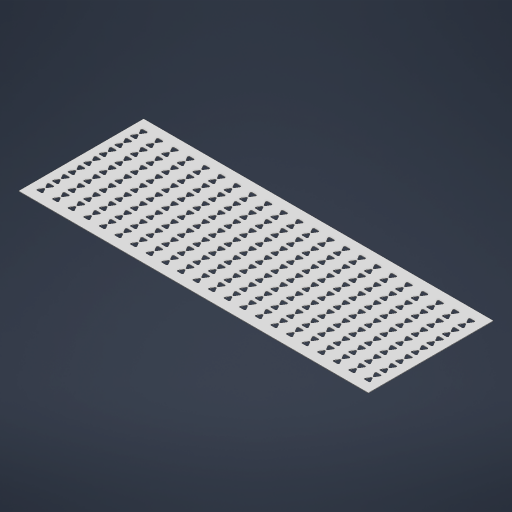
# Autodesk Inventor part: BellyPan
Saved by Autodesk Inventor 2023 (Build 270158000, 158)
## iProperties
Created: 2022-04-16
Part Number: BellyPan
Material: Generic
Document SubType Name: Modeling
Designer: timmy
Density: 1 g/cm^3
Appearance: Default
Author: timmy
Autodesk Inventor part; units mm, degrees
(part 1 of 4)
ref_plane "YZ Plane" through (0, 0, 0) normal (1, 0, 0) x (0, 1, 0)
ref_plane "XZ Plane" through (0, 0, 0) normal (0, 1, 0) x (-1, 0, 0)
ref_plane "XY Plane" through (0, 0, 0) normal (0, 0, 1) x (1, 0, 0)
sketch "Sketch1" plane through (0, 0, 0) normal (0, 1, 0) x (-1, 0, 0)
  line L0 (0, 0) -> (1219.2, 0)
  line L1 (1219.2, 0) -> (1219.2, -436.0164)
  line L2 (1219.2, -436.0164) -> (0, -436.0164)
  line L3 (0, -436.0164) -> (0, 0)
  dimension "d0" = 1219.2
  dimension "d1" = 436.0164
  constraints: 8 end point, 2 parallel, 1 horizontal, 1 perpendicular
  measures "d0" distance of L1.end L2.end
  measures "d1" distance of L0.end L1.end
extrude "Extrusion1" add sketch "Sketch1" along normal blind 1.5875
sketch "Sketch2" plane through (0, 1.5875, 0) normal (0, 1, 0) x (1, 0, 0)
  line L0 (0, 436.0164) -> (-1219.2, 436.0164) projected
  line L1 (-1219.2, 436.0164) -> (-1219.2, 0) projected
  line L2 (-1219.2, 0) -> (0, 0) projected
  line L3 (0, 0) -> (0, 436.0164) projected
  line L4 (-1193.8, 410.6164) -> (-1193.8, 25.4)
  line L5 (-25.4, 410.6164) -> (-1193.8, 410.6164)
  line L6 (-1188.4934, 33.8582) -> (-1174.092, 33.8582)
  line L7 (-1171.3423, 38.6207) -> (-1178.5431, 51.0927)
  line L8 (-1184.0423, 51.0927) -> (-1191.2431, 38.6207)
  arc A0 (-1191.2431, 38.6207) -> (-1188.4934, 33.8582) centre (-1188.4934, 37.0332) ccw
  arc A1 (-1174.092, 33.8582) -> (-1171.3423, 38.6207) centre (-1174.092, 37.0332) ccw
  arc A2 (-1178.5431, 51.0927) -> (-1184.0423, 51.0927) centre (-1181.2927, 49.5052) ccw
  line L9 (-1188.3007, 76.2) -> (-1173.8993, 76.2)
  line L10 (-1171.1496, 71.4375) -> (-1178.3504, 58.9655)
  line L11 (-1183.8496, 58.9655) -> (-1191.0504, 71.4375)
  arc A3 (-1188.3007, 76.2) -> (-1191.0504, 71.4375) centre (-1188.3007, 73.025) ccw
  arc A4 (-1171.1496, 71.4375) -> (-1173.8993, 76.2) centre (-1173.8993, 73.025) ccw
  arc A5 (-1183.8496, 58.9655) -> (-1178.3504, 58.9655) centre (-1181.1, 60.553) ccw
  line L12 (-1183.8496, 113.3215) -> (-1191.0504, 125.7935)
  arc A6 (-1171.1496, 125.7935) -> (-1173.8993, 130.556) centre (-1173.8993, 127.381) ccw
  arc A7 (-1188.3007, 130.556) -> (-1191.0504, 125.7935) centre (-1188.3007, 127.381) ccw
  arc A8 (-1183.8496, 113.3215) -> (-1178.3504, 113.3215) centre (-1181.1, 114.909) ccw
  line L13 (-1171.1496, 125.7935) -> (-1178.3504, 113.3215)
  line L14 (-1188.3007, 130.556) -> (-1173.8993, 130.556)
  arc A9 (-1178.5431, 105.4487) -> (-1184.0423, 105.4487) centre (-1181.2927, 103.8612) ccw
  line L15 (-1171.3423, 92.9767) -> (-1178.5431, 105.4487)
  line L16 (-1184.0423, 105.4487) -> (-1191.2431, 92.9767)
  arc A10 (-1191.2431, 92.9767) -> (-1188.4934, 88.2142) centre (-1188.4934, 91.3892) ccw
  line L17 (-1188.4934, 88.2142) -> (-1174.092, 88.2142)
  arc A11 (-1174.092, 88.2142) -> (-1171.3423, 92.9767) centre (-1174.092, 91.3892) ccw
  line L18 (-1183.8496, 167.6775) -> (-1191.0504, 180.1495)
  arc A12 (-1171.1496, 180.1495) -> (-1173.8993, 184.912) centre (-1173.8993, 181.737) ccw
  arc A13 (-1188.3007, 184.912) -> (-1191.0504, 180.1495) centre (-1188.3007, 181.737) ccw
  arc A14 (-1183.8496, 167.6775) -> (-1178.3504, 167.6775) centre (-1181.1, 169.265) ccw
  line L19 (-1171.1496, 180.1495) -> (-1178.3504, 167.6775)
  line L20 (-1188.3007, 184.912) -> (-1173.8993, 184.912)
  arc A15 (-1178.5431, 159.8047) -> (-1184.0423, 159.8047) centre (-1181.2927, 158.2172) ccw
  line L21 (-1171.3423, 147.3327) -> (-1178.5431, 159.8047)
  line L22 (-1184.0423, 159.8047) -> (-1191.2431, 147.3327)
  arc A16 (-1191.2431, 147.3327) -> (-1188.4934, 142.5702) centre (-1188.4934, 145.7452) ccw
  line L23 (-1188.4934, 142.5702) -> (-1174.092, 142.5702)
  arc A17 (-1174.092, 142.5702) -> (-1171.3423, 147.3327) centre (-1174.092, 145.7452) ccw
  line L24 (-1183.8496, 222.0335) -> (-1191.0504, 234.5055)
  arc A18 (-1171.1496, 234.5055) -> (-1173.8993, 239.268) centre (-1173.8993, 236.093) ccw
  arc A19 (-1188.3007, 239.268) -> (-1191.0504, 234.5055) centre (-1188.3007, 236.093) ccw
  arc A20 (-1183.8496, 222.0335) -> (-1178.3504, 222.0335) centre (-1181.1, 223.621) ccw
  line L25 (-1171.1496, 234.5055) -> (-1178.3504, 222.0335)
  line L26 (-1188.3007, 239.268) -> (-1173.8993, 239.268)
  arc A21 (-1178.5431, 214.1607) -> (-1184.0423, 214.1607) centre (-1181.2927, 212.5732) ccw
  line L27 (-1171.3423, 201.6887) -> (-1178.5431, 214.1607)
  line L28 (-1184.0423, 214.1607) -> (-1191.2431, 201.6887)
  arc A22 (-1191.2431, 201.6887) -> (-1188.4934, 196.9262) centre (-1188.4934, 200.1012) ccw
  line L29 (-1188.4934, 196.9262) -> (-1174.092, 196.9262)
  arc A23 (-1174.092, 196.9262) -> (-1171.3423, 201.6887) centre (-1174.092, 200.1012) ccw
  line L30 (-1183.8496, 276.3895) -> (-1191.0504, 288.8615)
  arc A24 (-1171.1496, 288.8615) -> (-1173.8993, 293.624) centre (-1173.8993, 290.449) ccw
  arc A25 (-1188.3007, 293.624) -> (-1191.0504, 288.8615) centre (-1188.3007, 290.449) ccw
  arc A26 (-1183.8496, 276.3895) -> (-1178.3504, 276.3895) centre (-1181.1, 277.977) ccw
  line L31 (-1171.1496, 288.8615) -> (-1178.3504, 276.3895)
  line L32 (-1188.3007, 293.624) -> (-1173.8993, 293.624)
  arc A27 (-1178.5431, 268.5167) -> (-1184.0423, 268.5167) centre (-1181.2927, 266.9292) ccw
  line L33 (-1171.3423, 256.0447) -> (-1178.5431, 268.5167)
  line L34 (-1184.0423, 268.5167) -> (-1191.2431, 256.0447)
  arc A28 (-1191.2431, 256.0447) -> (-1188.4934, 251.2822) centre (-1188.4934, 254.4572) ccw
  line L35 (-1188.4934, 251.2822) -> (-1174.092, 251.2822)
  arc A29 (-1174.092, 251.2822) -> (-1171.3423, 256.0447) centre (-1174.092, 254.4572) ccw
  line L36 (-1183.8496, 330.7455) -> (-1191.0504, 343.2175)
  arc A30 (-1171.1496, 343.2175) -> (-1173.8993, 347.98) centre (-1173.8993, 344.805) ccw
  arc A31 (-1188.3007, 347.98) -> (-1191.0504, 343.2175) centre (-1188.3007, 344.805) ccw
  arc A32 (-1183.8496, 330.7455) -> (-1178.3504, 330.7455) centre (-1181.1, 332.333) ccw
  line L37 (-1171.1496, 343.2175) -> (-1178.3504, 330.7455)
  line L38 (-1188.3007, 347.98) -> (-1173.8993, 347.98)
  arc A33 (-1178.5431, 322.8727) -> (-1184.0423, 322.8727) centre (-1181.2927, 321.2852) ccw
  line L39 (-1171.3423, 310.4007) -> (-1178.5431, 322.8727)
  line L40 (-1184.0423, 322.8727) -> (-1191.2431, 310.4007)
  arc A34 (-1191.2431, 310.4007) -> (-1188.4934, 305.6382) centre (-1188.4934, 308.8132) ccw
  line L41 (-1188.4934, 305.6382) -> (-1174.092, 305.6382)
  arc A35 (-1174.092, 305.6382) -> (-1171.3423, 310.4007) centre (-1174.092, 308.8132) ccw
  line L42 (-1183.8496, 385.1015) -> (-1191.0504, 397.5735)
  arc A36 (-1171.1496, 397.5735) -> (-1173.8993, 402.336) centre (-1173.8993, 399.161) ccw
  arc A37 (-1188.3007, 402.336) -> (-1191.0504, 397.5735) centre (-1188.3007, 399.161) ccw
  arc A38 (-1183.8496, 385.1015) -> (-1178.3504, 385.1015) centre (-1181.1, 386.689) ccw
  line L43 (-1171.1496, 397.5735) -> (-1178.3504, 385.1015)
  line L44 (-1188.3007, 402.336) -> (-1173.8993, 402.336)
  arc A39 (-1178.5431, 377.2287) -> (-1184.0423, 377.2287) centre (-1181.2927, 375.6412) ccw
  line L45 (-1171.3423, 364.7567) -> (-1178.5431, 377.2287)
  line L46 (-1184.0423, 377.2287) -> (-1191.2431, 364.7567)
  arc A40 (-1191.2431, 364.7567) -> (-1188.4934, 359.9942) centre (-1188.4934, 363.1692) ccw
  line L47 (-1188.4934, 359.9942) -> (-1174.092, 359.9942)
  arc A41 (-1174.092, 359.9942) -> (-1171.3423, 364.7567) centre (-1174.092, 363.1692) ccw
  line L48 (-1129.4936, 58.9655) -> (-1136.6944, 71.4375)
  arc A42 (-1116.7936, 71.4375) -> (-1119.5433, 76.2) centre (-1119.5433, 73.025) ccw
  arc A43 (-1133.9447, 76.2) -> (-1136.6944, 71.4375) centre (-1133.9447, 73.025) ccw
  arc A44 (-1129.4936, 58.9655) -> (-1123.9944, 58.9655) centre (-1126.744, 60.553) ccw
  line L49 (-1116.7936, 71.4375) -> (-1123.9944, 58.9655)
  line L50 (-1133.9447, 76.2) -> (-1119.5433, 76.2)
  arc A45 (-1124.1871, 51.0927) -> (-1129.6863, 51.0927) centre (-1126.9367, 49.5052) ccw
  line L51 (-1116.9863, 38.6207) -> (-1124.1871, 51.0927)
  line L52 (-1129.6863, 51.0927) -> (-1136.8871, 38.6207)
  arc A46 (-1136.8871, 38.6207) -> (-1134.1374, 33.8582) centre (-1134.1374, 37.0332) ccw
  line L53 (-1134.1374, 33.8582) -> (-1119.736, 33.8582)
  arc A47 (-1119.736, 33.8582) -> (-1116.9863, 38.6207) centre (-1119.736, 37.0332) ccw
  line L54 (-1129.4936, 113.3215) -> (-1136.6944, 125.7935)
  arc A48 (-1116.7936, 125.7935) -> (-1119.5433, 130.556) centre (-1119.5433, 127.381) ccw
  arc A49 (-1133.9447, 130.556) -> (-1136.6944, 125.7935) centre (-1133.9447, 127.381) ccw
  arc A50 (-1129.4936, 113.3215) -> (-1123.9944, 113.3215) centre (-1126.744, 114.909) ccw
  line L55 (-1116.7936, 125.7935) -> (-1123.9944, 113.3215)
  line L56 (-1133.9447, 130.556) -> (-1119.5433, 130.556)
  arc A51 (-1124.1871, 105.4487) -> (-1129.6863, 105.4487) centre (-1126.9367, 103.8612) ccw
  line L57 (-1116.9863, 92.9767) -> (-1124.1871, 105.4487)
  line L58 (-1129.6863, 105.4487) -> (-1136.8871, 92.9767)
  arc A52 (-1136.8871, 92.9767) -> (-1134.1374, 88.2142) centre (-1134.1374, 91.3892) ccw
  line L59 (-1134.1374, 88.2142) -> (-1119.736, 88.2142)
  arc A53 (-1119.736, 88.2142) -> (-1116.9863, 92.9767) centre (-1119.736, 91.3892) ccw
  line L60 (-1129.4936, 167.6775) -> (-1136.6944, 180.1495)
  arc A54 (-1116.7936, 180.1495) -> (-1119.5433, 184.912) centre (-1119.5433, 181.737) ccw
  arc A55 (-1133.9447, 184.912) -> (-1136.6944, 180.1495) centre (-1133.9447, 181.737) ccw
  arc A56 (-1129.4936, 167.6775) -> (-1123.9944, 167.6775) centre (-1126.744, 169.265) ccw
  line L61 (-1116.7936, 180.1495) -> (-1123.9944, 167.6775)
  line L62 (-1133.9447, 184.912) -> (-1119.5433, 184.912)
  arc A57 (-1124.1871, 159.8047) -> (-1129.6863, 159.8047) centre (-1126.9367, 158.2172) ccw
  line L63 (-1116.9863, 147.3327) -> (-1124.1871, 159.8047)
  line L64 (-1129.6863, 159.8047) -> (-1136.8871, 147.3327)
  arc A58 (-1136.8871, 147.3327) -> (-1134.1374, 142.5702) centre (-1134.1374, 145.7452) ccw
  line L65 (-1134.1374, 142.5702) -> (-1119.736, 142.5702)
  arc A59 (-1119.736, 142.5702) -> (-1116.9863, 147.3327) centre (-1119.736, 145.7452) ccw
  line L66 (-1129.4936, 222.0335) -> (-1136.6944, 234.5055)
  arc A60 (-1116.7936, 234.5055) -> (-1119.5433, 239.268) centre (-1119.5433, 236.093) ccw
  arc A61 (-1133.9447, 239.268) -> (-1136.6944, 234.5055) centre (-1133.9447, 236.093) ccw
  arc A62 (-1129.4936, 222.0335) -> (-1123.9944, 222.0335) centre (-1126.744, 223.621) ccw
  line L67 (-1116.7936, 234.5055) -> (-1123.9944, 222.0335)
  line L68 (-1133.9447, 239.268) -> (-1119.5433, 239.268)
  arc A63 (-1124.1871, 214.1607) -> (-1129.6863, 214.1607) centre (-1126.9367, 212.5732) ccw
  line L69 (-1116.9863, 201.6887) -> (-1124.1871, 214.1607)
  line L70 (-1129.6863, 214.1607) -> (-1136.8871, 201.6887)
  arc A64 (-1136.8871, 201.6887) -> (-1134.1374, 196.9262) centre (-1134.1374, 200.1012) ccw
  line L71 (-1134.1374, 196.9262) -> (-1119.736, 196.9262)
  arc A65 (-1119.736, 196.9262) -> (-1116.9863, 201.6887) centre (-1119.736, 200.1012) ccw
  line L72 (-1129.4936, 276.3895) -> (-1136.6944, 288.8615)
  arc A66 (-1116.7936, 288.8615) -> (-1119.5433, 293.624) centre (-1119.5433, 290.449) ccw
  arc A67 (-1133.9447, 293.624) -> (-1136.6944, 288.8615) centre (-1133.9447, 290.449) ccw
  arc A68 (-1129.4936, 276.3895) -> (-1123.9944, 276.3895) centre (-1126.744, 277.977) ccw
  line L73 (-1116.7936, 288.8615) -> (-1123.9944, 276.3895)
  line L74 (-1133.9447, 293.624) -> (-1119.5433, 293.624)
  arc A69 (-1124.1871, 268.5167) -> (-1129.6863, 268.5167) centre (-1126.9367, 266.9292) ccw
  line L75 (-1116.9863, 256.0447) -> (-1124.1871, 268.5167)
  line L76 (-1129.6863, 268.5167) -> (-1136.8871, 256.0447)
  arc A70 (-1136.8871, 256.0447) -> (-1134.1374, 251.2822) centre (-1134.1374, 254.4572) ccw
  line L77 (-1134.1374, 251.2822) -> (-1119.736, 251.2822)
  arc A71 (-1119.736, 251.2822) -> (-1116.9863, 256.0447) centre (-1119.736, 254.4572) ccw
  line L78 (-1129.4936, 330.7455) -> (-1136.6944, 343.2175)
  arc A72 (-1116.7936, 343.2175) -> (-1119.5433, 347.98) centre (-1119.5433, 344.805) ccw
  arc A73 (-1133.9447, 347.98) -> (-1136.6944, 343.2175) centre (-1133.9447, 344.805) ccw
  arc A74 (-1129.4936, 330.7455) -> (-1123.9944, 330.7455) centre (-1126.744, 332.333) ccw
  line L79 (-1116.7936, 343.2175) -> (-1123.9944, 330.7455)
  line L80 (-1133.9447, 347.98) -> (-1119.5433, 347.98)
  arc A75 (-1124.1871, 322.8727) -> (-1129.6863, 322.8727) centre (-1126.9367, 321.2852) ccw
  line L81 (-1116.9863, 310.4007) -> (-1124.1871, 322.8727)
  line L82 (-1129.6863, 322.8727) -> (-1136.8871, 310.4007)
  arc A76 (-1136.8871, 310.4007) -> (-1134.1374, 305.6382) centre (-1134.1374, 308.8132) ccw
  line L83 (-1134.1374, 305.6382) -> (-1119.736, 305.6382)
  arc A77 (-1119.736, 305.6382) -> (-1116.9863, 310.4007) centre (-1119.736, 308.8132) ccw
  line L84 (-1129.4936, 385.1015) -> (-1136.6944, 397.5735)
  arc A78 (-1116.7936, 397.5735) -> (-1119.5433, 402.336) centre (-1119.5433, 399.161) ccw
  arc A79 (-1133.9447, 402.336) -> (-1136.6944, 397.5735) centre (-1133.9447, 399.161) ccw
  arc A80 (-1129.4936, 385.1015) -> (-1123.9944, 385.1015) centre (-1126.744, 386.689) ccw
  line L85 (-1116.7936, 397.5735) -> (-1123.9944, 385.1015)
  line L86 (-1133.9447, 402.336) -> (-1119.5433, 402.336)
  arc A81 (-1124.1871, 377.2287) -> (-1129.6863, 377.2287) centre (-1126.9367, 375.6412) ccw
  line L87 (-1116.9863, 364.7567) -> (-1124.1871, 377.2287)
  line L88 (-1129.6863, 377.2287) -> (-1136.8871, 364.7567)
  arc A82 (-1136.8871, 364.7567) -> (-1134.1374, 359.9942) centre (-1134.1374, 363.1692) ccw
  line L89 (-1134.1374, 359.9942) -> (-1119.736, 359.9942)
  arc A83 (-1119.736, 359.9942) -> (-1116.9863, 364.7567) centre (-1119.736, 363.1692) ccw
  line L90 (-1075.1376, 58.9655) -> (-1082.3384, 71.4375)
  arc A84 (-1062.4376, 71.4375) -> (-1065.1873, 76.2) centre (-1065.1873, 73.025) ccw
  arc A85 (-1079.5887, 76.2) -> (-1082.3384, 71.4375) centre (-1079.5887, 73.025) ccw
  arc A86 (-1075.1376, 58.9655) -> (-1069.6384, 58.9655) centre (-1072.388, 60.553) ccw
  line L91 (-1062.4376, 71.4375) -> (-1069.6384, 58.9655)
  line L92 (-1079.5887, 76.2) -> (-1065.1873, 76.2)
  arc A87 (-1069.8311, 51.0927) -> (-1075.3303, 51.0927) centre (-1072.5807, 49.5052) ccw
  line L93 (-1062.6303, 38.6207) -> (-1069.8311, 51.0927)
  line L94 (-1075.3303, 51.0927) -> (-1082.5311, 38.6207)
  arc A88 (-1082.5311, 38.6207) -> (-1079.7814, 33.8582) centre (-1079.7814, 37.0332) ccw
  line L95 (-1079.7814, 33.8582) -> (-1065.38, 33.8582)
  arc A89 (-1065.38, 33.8582) -> (-1062.6303, 38.6207) centre (-1065.38, 37.0332) ccw
  line L96 (-1075.1376, 113.3215) -> (-1082.3384, 125.7935)
  arc A90 (-1062.4376, 125.7935) -> (-1065.1873, 130.556) centre (-1065.1873, 127.381) ccw
  arc A91 (-1079.5887, 130.556) -> (-1082.3384, 125.7935) centre (-1079.5887, 127.381) ccw
  arc A92 (-1075.1376, 113.3215) -> (-1069.6384, 113.3215) centre (-1072.388, 114.909) ccw
  line L97 (-1062.4376, 125.7935) -> (-1069.6384, 113.3215)
  line L98 (-1079.5887, 130.556) -> (-1065.1873, 130.556)
  arc A93 (-1069.8311, 105.4487) -> (-1075.3303, 105.4487) centre (-1072.5807, 103.8612) ccw
  line L99 (-1062.6303, 92.9767) -> (-1069.8311, 105.4487)
  line L100 (-1075.3303, 105.4487) -> (-1082.5311, 92.9767)
  arc A94 (-1082.5311, 92.9767) -> (-1079.7814, 88.2142) centre (-1079.7814, 91.3892) ccw
  line L101 (-1079.7814, 88.2142) -> (-1065.38, 88.2142)
  arc A95 (-1065.38, 88.2142) -> (-1062.6303, 92.9767) centre (-1065.38, 91.3892) ccw
  line L102 (-1075.1376, 167.6775) -> (-1082.3384, 180.1495)
  arc A96 (-1062.4376, 180.1495) -> (-1065.1873, 184.912) centre (-1065.1873, 181.737) ccw
  arc A97 (-1079.5887, 184.912) -> (-1082.3384, 180.1495) centre (-1079.5887, 181.737) ccw
  arc A98 (-1075.1376, 167.6775) -> (-1069.6384, 167.6775) centre (-1072.388, 169.265) ccw
  line L103 (-1062.4376, 180.1495) -> (-1069.6384, 167.6775)
  line L104 (-1079.5887, 184.912) -> (-1065.1873, 184.912)
  arc A99 (-1069.8311, 159.8047) -> (-1075.3303, 159.8047) centre (-1072.5807, 158.2172) ccw
  line L105 (-1062.6303, 147.3327) -> (-1069.8311, 159.8047)
  line L106 (-1075.3303, 159.8047) -> (-1082.5311, 147.3327)
  arc A100 (-1082.5311, 147.3327) -> (-1079.7814, 142.5702) centre (-1079.7814, 145.7452) ccw
  line L107 (-1079.7814, 142.5702) -> (-1065.38, 142.5702)
  arc A101 (-1065.38, 142.5702) -> (-1062.6303, 147.3327) centre (-1065.38, 145.7452) ccw
  line L108 (-1075.1376, 222.0335) -> (-1082.3384, 234.5055)
  arc A102 (-1062.4376, 234.5055) -> (-1065.1873, 239.268) centre (-1065.1873, 236.093) ccw
  arc A103 (-1079.5887, 239.268) -> (-1082.3384, 234.5055) centre (-1079.5887, 236.093) ccw
  arc A104 (-1075.1376, 222.0335) -> (-1069.6384, 222.0335) centre (-1072.388, 223.621) ccw
  line L109 (-1062.4376, 234.5055) -> (-1069.6384, 222.0335)
  line L110 (-1079.5887, 239.268) -> (-1065.1873, 239.268)
  arc A105 (-1069.8311, 214.1607) -> (-1075.3303, 214.1607) centre (-1072.5807, 212.5732) ccw
  line L111 (-1062.6303, 201.6887) -> (-1069.8311, 214.1607)
  line L112 (-1075.3303, 214.1607) -> (-1082.5311, 201.6887)
  arc A106 (-1082.5311, 201.6887) -> (-1079.7814, 196.9262) centre (-1079.7814, 200.1012) ccw
  line L113 (-1079.7814, 196.9262) -> (-1065.38, 196.9262)
  arc A107 (-1065.38, 196.9262) -> (-1062.6303, 201.6887) centre (-1065.38, 200.1012) ccw
  line L114 (-1075.1376, 276.3895) -> (-1082.3384, 288.8615)
  arc A108 (-1062.4376, 288.8615) -> (-1065.1873, 293.624) centre (-1065.1873, 290.449) ccw
  arc A109 (-1079.5887, 293.624) -> (-1082.3384, 288.8615) centre (-1079.5887, 290.449) ccw
  arc A110 (-1075.1376, 276.3895) -> (-1069.6384, 276.3895) centre (-1072.388, 277.977) ccw
  line L115 (-1062.4376, 288.8615) -> (-1069.6384, 276.3895)
  line L116 (-1079.5887, 293.624) -> (-1065.1873, 293.624)
  arc A111 (-1069.8311, 268.5167) -> (-1075.3303, 268.5167) centre (-1072.5807, 266.9292) ccw
  line L117 (-1062.6303, 256.0447) -> (-1069.8311, 268.5167)
  line L118 (-1075.3303, 268.5167) -> (-1082.5311, 256.0447)
  arc A112 (-1082.5311, 256.0447) -> (-1079.7814, 251.2822) centre (-1079.7814, 254.4572) ccw
  line L119 (-1079.7814, 251.2822) -> (-1065.38, 251.2822)
  arc A113 (-1065.38, 251.2822) -> (-1062.6303, 256.0447) centre (-1065.38, 254.4572) ccw
  line L120 (-1075.1376, 330.7455) -> (-1082.3384, 343.2175)
  arc A114 (-1062.4376, 343.2175) -> (-1065.1873, 347.98) centre (-1065.1873, 344.805) ccw
  arc A115 (-1079.5887, 347.98) -> (-1082.3384, 343.2175) centre (-1079.5887, 344.805) ccw
  arc A116 (-1075.1376, 330.7455) -> (-1069.6384, 330.7455) centre (-1072.388, 332.333) ccw
  line L121 (-1062.4376, 343.2175) -> (-1069.6384, 330.7455)
  line L122 (-1079.5887, 347.98) -> (-1065.1873, 347.98)
  arc A117 (-1069.8311, 322.8727) -> (-1075.3303, 322.8727) centre (-1072.5807, 321.2852) ccw
  line L123 (-1062.6303, 310.4007) -> (-1069.8311, 322.8727)
  line L124 (-1075.3303, 322.8727) -> (-1082.5311, 310.4007)
  arc A118 (-1082.5311, 310.4007) -> (-1079.7814, 305.6382) centre (-1079.7814, 308.8132) ccw
  line L125 (-1079.7814, 305.6382) -> (-1065.38, 305.6382)
  arc A119 (-1065.38, 305.6382) -> (-1062.6303, 310.4007) centre (-1065.38, 308.8132) ccw
  line L126 (-1075.1376, 385.1015) -> (-1082.3384, 397.5735)
  arc A120 (-1062.4376, 397.5735) -> (-1065.1873, 402.336) centre (-1065.1873, 399.161) ccw
  arc A121 (-1079.5887, 402.336) -> (-1082.3384, 397.5735) centre (-1079.5887, 399.161) ccw
  arc A122 (-1075.1376, 385.1015) -> (-1069.6384, 385.1015) centre (-1072.388, 386.689) ccw
  line L127 (-1062.4376, 397.5735) -> (-1069.6384, 385.1015)
  line L128 (-1079.5887, 402.336) -> (-1065.1873, 402.336)
  arc A123 (-1069.8311, 377.2287) -> (-1075.3303, 377.2287) centre (-1072.5807, 375.6412) ccw
  line L129 (-1062.6303, 364.7567) -> (-1069.8311, 377.2287)
  line L130 (-1075.3303, 377.2287) -> (-1082.5311, 364.7567)
  arc A124 (-1082.5311, 364.7567) -> (-1079.7814, 359.9942) centre (-1079.7814, 363.1692) ccw
  line L131 (-1079.7814, 359.9942) -> (-1065.38, 359.9942)
  arc A125 (-1065.38, 359.9942) -> (-1062.6303, 364.7567) centre (-1065.38, 363.1692) ccw
  line L132 (-1020.7816, 58.9655) -> (-1027.9824, 71.4375)
  arc A126 (-1008.0816, 71.4375) -> (-1010.8313, 76.2) centre (-1010.8313, 73.025) ccw
  arc A127 (-1025.2327, 76.2) -> (-1027.9824, 71.4375) centre (-1025.2327, 73.025) ccw
  arc A128 (-1020.7816, 58.9655) -> (-1015.2824, 58.9655) centre (-1018.032, 60.553) ccw
  line L133 (-1008.0816, 71.4375) -> (-1015.2824, 58.9655)
  line L134 (-1025.2327, 76.2) -> (-1010.8313, 76.2)
  arc A129 (-1015.4751, 51.0927) -> (-1020.9743, 51.0927) centre (-1018.2247, 49.5052) ccw
  line L135 (-1008.2743, 38.6207) -> (-1015.4751, 51.0927)
  line L136 (-1020.9743, 51.0927) -> (-1028.1751, 38.6207)
  arc A130 (-1028.1751, 38.6207) -> (-1025.4254, 33.8582) centre (-1025.4254, 37.0332) ccw
  line L137 (-1025.4254, 33.8582) -> (-1011.024, 33.8582)
  arc A131 (-1011.024, 33.8582) -> (-1008.2743, 38.6207) centre (-1011.024, 37.0332) ccw
  line L138 (-1020.7816, 113.3215) -> (-1027.9824, 125.7935)
  arc A132 (-1008.0816, 125.7935) -> (-1010.8313, 130.556) centre (-1010.8313, 127.381) ccw
  arc A133 (-1025.2327, 130.556) -> (-1027.9824, 125.7935) centre (-1025.2327, 127.381) ccw
  arc A134 (-1020.7816, 113.3215) -> (-1015.2824, 113.3215) centre (-1018.032, 114.909) ccw
  line L139 (-1008.0816, 125.7935) -> (-1015.2824, 113.3215)
  line L140 (-1025.2327, 130.556) -> (-1010.8313, 130.556)
  arc A135 (-1015.4751, 105.4487) -> (-1020.9743, 105.4487) centre (-1018.2247, 103.8612) ccw
  line L141 (-1008.2743, 92.9767) -> (-1015.4751, 105.4487)
  line L142 (-1020.9743, 105.4487) -> (-1028.1751, 92.9767)
  arc A136 (-1028.1751, 92.9767) -> (-1025.4254, 88.2142) centre (-1025.4254, 91.3892) ccw
  line L143 (-1025.4254, 88.2142) -> (-1011.024, 88.2142)
  arc A137 (-1011.024, 88.2142) -> (-1008.2743, 92.9767) centre (-1011.024, 91.3892) ccw
  line L144 (-1020.7816, 167.6775) -> (-1027.9824, 180.1495)
  arc A138 (-1008.0816, 180.1495) -> (-1010.8313, 184.912) centre (-1010.8313, 181.737) ccw
  arc A139 (-1025.2327, 184.912) -> (-1027.9824, 180.1495) centre (-1025.2327, 181.737) ccw
  arc A140 (-1020.7816, 167.6775) -> (-1015.2824, 167.6775) centre (-1018.032, 169.265) ccw
  line L145 (-1008.0816, 180.1495) -> (-1015.2824, 167.6775)
  line L146 (-1025.2327, 184.912) -> (-1010.8313, 184.912)
  arc A141 (-1015.4751, 159.8047) -> (-1020.9743, 159.8047) centre (-1018.2247, 158.2172) ccw
  line L147 (-1008.2743, 147.3327) -> (-1015.4751, 159.8047)
  line L148 (-1020.9743, 159.8047) -> (-1028.1751, 147.3327)
  arc A142 (-1028.1751, 147.3327) -> (-1025.4254, 142.5702) centre (-1025.4254, 145.7452) ccw
  line L149 (-1025.4254, 142.5702) -> (-1011.024, 142.5702)
  arc A143 (-1011.024, 142.5702) -> (-1008.2743, 147.3327) centre (-1011.024, 145.7452) ccw
  line L150 (-1020.7816, 222.0335) -> (-1027.9824, 234.5055)
  arc A144 (-1008.0816, 234.5055) -> (-1010.8313, 239.268) centre (-1010.8313, 236.093) ccw
  arc A145 (-1025.2327, 239.268) -> (-1027.9824, 234.5055) centre (-1025.2327, 236.093) ccw
  arc A146 (-1020.7816, 222.0335) -> (-1015.2824, 222.0335) centre (-1018.032, 223.621) ccw
  line L151 (-1008.0816, 234.5055) -> (-1015.2824, 222.0335)
  line L152 (-1025.2327, 239.268) -> (-1010.8313, 239.268)
  arc A147 (-1015.4751, 214.1607) -> (-1020.9743, 214.1607) centre (-1018.2247, 212.5732) ccw
  line L153 (-1008.2743, 201.6887) -> (-1015.4751, 214.1607)
  line L154 (-1020.9743, 214.1607) -> (-1028.1751, 201.6887)
  arc A148 (-1028.1751, 201.6887) -> (-1025.4254, 196.9262) centre (-1025.4254, 200.1012) ccw
  line L155 (-1025.4254, 196.9262) -> (-1011.024, 196.9262)
  arc A149 (-1011.024, 196.9262) -> (-1008.2743, 201.6887) centre (-1011.024, 200.1012) ccw
  line L156 (-1020.7816, 276.3895) -> (-1027.9824, 288.8615)
  arc A150 (-1008.0816, 288.8615) -> (-1010.8313, 293.624) centre (-1010.8313, 290.449) ccw
  arc A151 (-1025.2327, 293.624) -> (-1027.9824, 288.8615) centre (-1025.2327, 290.449) ccw
  arc A152 (-1020.7816, 276.3895) -> (-1015.2824, 276.3895) centre (-1018.032, 277.977) ccw
  line L157 (-1008.0816, 288.8615) -> (-1015.2824, 276.3895)
  line L158 (-1025.2327, 293.624) -> (-1010.8313, 293.624)
  arc A153 (-1015.4751, 268.5167) -> (-1020.9743, 268.5167) centre (-1018.2247, 266.9292) ccw
  line L159 (-1008.2743, 256.0447) -> (-1015.4751, 268.5167)
  line L160 (-1020.9743, 268.5167) -> (-1028.1751, 256.0447)
  arc A154 (-1028.1751, 256.0447) -> (-1025.4254, 251.2822) centre (-1025.4254, 254.4572) ccw
  line L161 (-1025.4254, 251.2822) -> (-1011.024, 251.2822)
  arc A155 (-1011.024, 251.2822) -> (-1008.2743, 256.0447) centre (-1011.024, 254.4572) ccw
  line L162 (-1020.7816, 330.7455) -> (-1027.9824, 343.2175)
  arc A156 (-1008.0816, 343.2175) -> (-1010.8313, 347.98) centre (-1010.8313, 344.805) ccw
  arc A157 (-1025.2327, 347.98) -> (-1027.9824, 343.2175) centre (-1025.2327, 344.805) ccw
  arc A158 (-1020.7816, 330.7455) -> (-1015.2824, 330.7455) centre (-1018.032, 332.333) ccw
  line L163 (-1008.0816, 343.2175) -> (-1015.2824, 330.7455)
  line L164 (-1025.2327, 347.98) -> (-1010.8313, 347.98)
  arc A159 (-1015.4751, 322.8727) -> (-1020.9743, 322.8727) centre (-1018.2247, 321.2852) ccw
  line L165 (-1008.2743, 310.4007) -> (-1015.4751, 322.8727)
  line L166 (-1020.9743, 322.8727) -> (-1028.1751, 310.4007)
  arc A160 (-1028.1751, 310.4007) -> (-1025.4254, 305.6382) centre (-1025.4254, 308.8132) ccw
  line L167 (-1025.4254, 305.6382) -> (-1011.024, 305.6382)
  arc A161 (-1011.024, 305.6382) -> (-1008.2743, 310.4007) centre (-1011.024, 308.8132) ccw
  line L168 (-1020.7816, 385.1015) -> (-1027.9824, 397.5735)
  arc A162 (-1008.0816, 397.5735) -> (-1010.8313, 402.336) centre (-1010.8313, 399.161) ccw
  arc A163 (-1025.2327, 402.336) -> (-1027.9824, 397.5735) centre (-1025.2327, 399.161) ccw
  arc A164 (-1020.7816, 385.1015) -> (-1015.2824, 385.1015) centre (-1018.032, 386.689) ccw
  line L169 (-1008.0816, 397.5735) -> (-1015.2824, 385.1015)
  line L170 (-1025.2327, 402.336) -> (-1010.8313, 402.336)
  arc A165 (-1015.4751, 377.2287) -> (-1020.9743, 377.2287) centre (-1018.2247, 375.6412) ccw
  line L171 (-1008.2743, 364.7567) -> (-1015.4751, 377.2287)
  line L172 (-1020.9743, 377.2287) -> (-1028.1751, 364.7567)
  arc A166 (-1028.1751, 364.7567) -> (-1025.4254, 359.9942) centre (-1025.4254, 363.1692) ccw
  line L173 (-1025.4254, 359.9942) -> (-1011.024, 359.9942)
  arc A167 (-1011.024, 359.9942) -> (-1008.2743, 364.7567) centre (-1011.024, 363.1692) ccw
  line L174 (-966.4256, 58.9655) -> (-973.6264, 71.4375)
  arc A168 (-953.7256, 71.4375) -> (-956.4753, 76.2) centre (-956.4753, 73.025) ccw
  arc A169 (-970.8767, 76.2) -> (-973.6264, 71.4375) centre (-970.8767, 73.025) ccw
  arc A170 (-966.4256, 58.9655) -> (-960.9264, 58.9655) centre (-963.676, 60.553) ccw
  line L175 (-953.7256, 71.4375) -> (-960.9264, 58.9655)
  line L176 (-970.8767, 76.2) -> (-956.4753, 76.2)
  arc A171 (-961.1191, 51.0927) -> (-966.6183, 51.0927) centre (-963.8687, 49.5052) ccw
  line L177 (-953.9183, 38.6207) -> (-961.1191, 51.0927)
  line L178 (-966.6183, 51.0927) -> (-973.8191, 38.6207)
  arc A172 (-973.8191, 38.6207) -> (-971.0694, 33.8582) centre (-971.0694, 37.0332) ccw
  line L179 (-971.0694, 33.8582) -> (-956.668, 33.8582)
  arc A173 (-956.668, 33.8582) -> (-953.9183, 38.6207) centre (-956.668, 37.0332) ccw
  line L180 (-966.4256, 113.3215) -> (-973.6264, 125.7935)
  arc A174 (-953.7256, 125.7935) -> (-956.4753, 130.556) centre (-956.4753, 127.381) ccw
  arc A175 (-970.8767, 130.556) -> (-973.6264, 125.7935) centre (-970.8767, 127.381) ccw
  arc A176 (-966.4256, 113.3215) -> (-960.9264, 113.3215) centre (-963.676, 114.909) ccw
  line L181 (-953.7256, 125.7935) -> (-960.9264, 113.3215)
  line L182 (-970.8767, 130.556) -> (-956.4753, 130.556)
  arc A177 (-961.1191, 105.4487) -> (-966.6183, 105.4487) centre (-963.8687, 103.8612) ccw
  line L183 (-953.9183, 92.9767) -> (-961.1191, 105.4487)
  line L184 (-966.6183, 105.4487) -> (-973.8191, 92.9767)
  arc A178 (-973.8191, 92.9767) -> (-971.0694, 88.2142) centre (-971.0694, 91.3892) ccw
  line L185 (-971.0694, 88.2142) -> (-956.668, 88.2142)
  arc A179 (-956.668, 88.2142) -> (-953.9183, 92.9767) centre (-956.668, 91.3892) ccw
  line L186 (-966.4256, 167.6775) -> (-973.6264, 180.1495)
  arc A180 (-953.7256, 180.1495) -> (-956.4753, 184.912) centre (-956.4753, 181.737) ccw
  arc A181 (-970.8767, 184.912) -> (-973.6264, 180.1495) centre (-970.8767, 181.737) ccw
  arc A182 (-966.4256, 167.6775) -> (-960.9264, 167.6775) centre (-963.676, 169.265) ccw
  line L187 (-953.7256, 180.1495) -> (-960.9264, 167.6775)
  line L188 (-970.8767, 184.912) -> (-956.4753, 184.912)
  arc A183 (-961.1191, 159.8047) -> (-966.6183, 159.8047) centre (-963.8687, 158.2172) ccw
  line L189 (-953.9183, 147.3327) -> (-961.1191, 159.8047)
  line L190 (-966.6183, 159.8047) -> (-973.8191, 147.3327)
  arc A184 (-973.8191, 147.3327) -> (-971.0694, 142.5702) centre (-971.0694, 145.7452) ccw
  line L191 (-971.0694, 142.5702) -> (-956.668, 142.5702)
  arc A185 (-956.668, 142.5702) -> (-953.9183, 147.3327) centre (-956.668, 145.7452) ccw
  line L192 (-966.4256, 222.0335) -> (-973.6264, 234.5055)
  arc A186 (-953.7256, 234.5055) -> (-956.4753, 239.268) centre (-956.4753, 236.093) ccw
  arc A187 (-970.8767, 239.268) -> (-973.6264, 234.5055) centre (-970.8767, 236.093) ccw
  arc A188 (-966.4256, 222.0335) -> (-960.9264, 222.0335) centre (-963.676, 223.621) ccw
  line L193 (-953.7256, 234.5055) -> (-960.9264, 222.0335)
  line L194 (-970.8767, 239.268) -> (-956.4753, 239.268)
  arc A189 (-961.1191, 214.1607) -> (-966.6183, 214.1607) centre (-963.8687, 212.5732) ccw
  line L195 (-953.9183, 201.6887) -> (-961.1191, 214.1607)
  line L196 (-966.6183, 214.1607) -> (-973.8191, 201.6887)
  arc A190 (-973.8191, 201.6887) -> (-971.0694, 196.9262) centre (-971.0694, 200.1012) ccw
  line L197 (-971.0694, 196.9262) -> (-956.668, 196.9262)
  arc A191 (-956.668, 196.9262) -> (-953.9183, 201.6887) centre (-956.668, 200.1012) ccw
  line L198 (-966.4256, 276.3895) -> (-973.6264, 288.8615)
  arc A192 (-953.7256, 288.8615) -> (-956.4753, 293.624) centre (-956.4753, 290.449) ccw
  arc A193 (-970.8767, 293.624) -> (-973.6264, 288.8615) centre (-970.8767, 290.449) ccw
  arc A194 (-966.4256, 276.3895) -> (-960.9264, 276.3895) centre (-963.676, 277.977) ccw
  line L199 (-953.7256, 288.8615) -> (-960.9264, 276.3895)
  line L200 (-970.8767, 293.624) -> (-956.4753, 293.624)
  arc A195 (-961.1191, 268.5167) -> (-966.6183, 268.5167) centre (-963.8687, 266.9292) ccw
  line L201 (-953.9183, 256.0447) -> (-961.1191, 268.5167)
  line L202 (-966.6183, 268.5167) -> (-973.8191, 256.0447)
  arc A196 (-973.8191, 256.0447) -> (-971.0694, 251.2822) centre (-971.0694, 254.4572) ccw
  line L203 (-971.0694, 251.2822) -> (-956.668, 251.2822)
  arc A197 (-956.668, 251.2822) -> (-953.9183, 256.0447) centre (-956.668, 254.4572) ccw
  line L204 (-966.4256, 330.7455) -> (-973.6264, 343.2175)
  arc A198 (-953.7256, 343.2175) -> (-956.4753, 347.98) centre (-956.4753, 344.805) ccw
  arc A199 (-970.8767, 347.98) -> (-973.6264, 343.2175) centre (-970.8767, 344.805) ccw
  arc A200 (-966.4256, 330.7455) -> (-960.9264, 330.7455) centre (-963.676, 332.333) ccw
  line L205 (-953.7256, 343.2175) -> (-960.9264, 330.7455)
  line L206 (-970.8767, 347.98) -> (-956.4753, 347.98)
  arc A201 (-961.1191, 322.8727) -> (-966.6183, 322.8727) centre (-963.8687, 321.2852) ccw
  line L207 (-953.9183, 310.4007) -> (-961.1191, 322.8727)
  line L208 (-966.6183, 322.8727) -> (-973.8191, 310.4007)
  arc A202 (-973.8191, 310.4007) -> (-971.0694, 305.6382) centre (-971.0694, 308.8132) ccw
  line L209 (-971.0694, 305.6382) -> (-956.668, 305.6382)
  arc A203 (-956.668, 305.6382) -> (-953.9183, 310.4007) centre (-956.668, 308.8132) ccw
  line L210 (-966.4256, 385.1015) -> (-973.6264, 397.5735)
  arc A204 (-953.7256, 397.5735) -> (-956.4753, 402.336) centre (-956.4753, 399.161) ccw
  arc A205 (-970.8767, 402.336) -> (-973.6264, 397.5735) centre (-970.8767, 399.161) ccw
  arc A206 (-966.4256, 385.1015) -> (-960.9264, 385.1015) centre (-963.676, 386.689) ccw
  line L211 (-953.7256, 397.5735) -> (-960.9264, 385.1015)
  line L212 (-970.8767, 402.336) -> (-956.4753, 402.336)
  arc A207 (-961.1191, 377.2287) -> (-966.6183, 377.2287) centre (-963.8687, 375.6412) ccw
  line L213 (-953.9183, 364.7567) -> (-961.1191, 377.2287)
  line L214 (-966.6183, 377.2287) -> (-973.8191, 364.7567)
  arc A208 (-973.8191, 364.7567) -> (-971.0694, 359.9942) centre (-971.0694, 363.1692) ccw
  line L215 (-971.0694, 359.9942) -> (-956.668, 359.9942)
  arc A209 (-956.668, 359.9942) -> (-953.9183, 364.7567) centre (-956.668, 363.1692) ccw
  line L216 (-912.0696, 58.9655) -> (-919.2704, 71.4375)
  arc A210 (-899.3696, 71.4375) -> (-902.1193, 76.2) centre (-902.1193, 73.025) ccw
  arc A211 (-916.5207, 76.2) -> (-919.2704, 71.4375) centre (-916.5207, 73.025) ccw
  arc A212 (-912.0696, 58.9655) -> (-906.5704, 58.9655) centre (-909.32, 60.553) ccw
  line L217 (-899.3696, 71.4375) -> (-906.5704, 58.9655)
  line L218 (-916.5207, 76.2) -> (-902.1193, 76.2)
  arc A213 (-906.7631, 51.0927) -> (-912.2623, 51.0927) centre (-909.5127, 49.5052) ccw
  line L219 (-899.5623, 38.6207) -> (-906.7631, 51.0927)
  line L220 (-912.2623, 51.0927) -> (-919.4631, 38.6207)
  arc A214 (-919.4631, 38.6207) -> (-916.7134, 33.8582) centre (-916.7134, 37.0332) ccw
  line L221 (-916.7134, 33.8582) -> (-902.312, 33.8582)
  arc A215 (-902.312, 33.8582) -> (-899.5623, 38.6207) centre (-902.312, 37.0332) ccw
  line L222 (-912.0696, 113.3215) -> (-919.2704, 125.7935)
  arc A216 (-899.3696, 125.7935) -> (-902.1193, 130.556) centre (-902.1193, 127.381) ccw
  arc A217 (-916.5207, 130.556) -> (-919.2704, 125.7935) centre (-916.5207, 127.381) ccw
  arc A218 (-912.0696, 113.3215) -> (-906.5704, 113.3215) centre (-909.32, 114.909) ccw
  line L223 (-899.3696, 125.7935) -> (-906.5704, 113.3215)
  line L224 (-916.5207, 130.556) -> (-902.1193, 130.556)
  arc A219 (-906.7631, 105.4487) -> (-912.2623, 105.4487) centre (-909.5127, 103.8612) ccw
  line L225 (-899.5623, 92.9767) -> (-906.7631, 105.4487)
  line L226 (-912.2623, 105.4487) -> (-919.4631, 92.9767)
  arc A220 (-919.4631, 92.9767) -> (-916.7134, 88.2142) centre (-916.7134, 91.3892) ccw
  line L227 (-916.7134, 88.2142) -> (-902.312, 88.2142)
  arc A221 (-902.312, 88.2142) -> (-899.5623, 92.9767) centre (-902.312, 91.3892) ccw
  line L228 (-912.0696, 167.6775) -> (-919.2704, 180.1495)
  arc A222 (-899.3696, 180.1495) -> (-902.1193, 184.912) centre (-902.1193, 181.737) ccw
  arc A223 (-916.5207, 184.912) -> (-919.2704, 180.1495) centre (-916.5207, 181.737) ccw
  arc A224 (-912.0696, 167.6775) -> (-906.5704, 167.6775) centre (-909.32, 169.265) ccw
  line L229 (-899.3696, 180.1495) -> (-906.5704, 167.6775)
  line L230 (-916.5207, 184.912) -> (-902.1193, 184.912)
  arc A225 (-906.7631, 159.8047) -> (-912.2623, 159.8047) centre (-909.5127, 158.2172) ccw
  line L231 (-899.5623, 147.3327) -> (-906.7631, 159.8047)
  line L232 (-912.2623, 159.8047) -> (-919.4631, 147.3327)
  arc A226 (-919.4631, 147.3327) -> (-916.7134, 142.5702) centre (-916.7134, 145.7452) ccw
  line L233 (-916.7134, 142.5702) -> (-902.312, 142.5702)
  arc A227 (-902.312, 142.5702) -> (-899.5623, 147.3327) centre (-902.312, 145.7452) ccw
  line L234 (-912.0696, 222.0335) -> (-919.2704, 234.5055)
  arc A228 (-899.3696, 234.5055) -> (-902.1193, 239.268) centre (-902.1193, 236.093) ccw
  arc A229 (-916.5207, 239.268) -> (-919.2704, 234.5055) centre (-916.5207, 236.093) ccw
  arc A230 (-912.0696, 222.0335) -> (-906.5704, 222.0335) centre (-909.32, 223.621) ccw
  line L235 (-899.3696, 234.5055) -> (-906.5704, 222.0335)
  line L236 (-916.5207, 239.268) -> (-902.1193, 239.268)
  arc A231 (-906.7631, 214.1607) -> (-912.2623, 214.1607) centre (-909.5127, 212.5732) ccw
  line L237 (-899.5623, 201.6887) -> (-906.7631, 214.1607)
  line L238 (-912.2623, 214.1607) -> (-919.4631, 201.6887)
  arc A232 (-919.4631, 201.6887) -> (-916.7134, 196.9262) centre (-916.7134, 200.1012) ccw
  line L239 (-916.7134, 196.9262) -> (-902.312, 196.9262)
  arc A233 (-902.312, 196.9262) -> (-899.5623, 201.6887) centre (-902.312, 200.1012) ccw
  line L240 (-912.0696, 276.3895) -> (-919.2704, 288.8615)
  arc A234 (-899.3696, 288.8615) -> (-902.1193, 293.624) centre (-902.1193, 290.449) ccw
  arc A235 (-916.5207, 293.624) -> (-919.2704, 288.8615) centre (-916.5207, 290.449) ccw
  arc A236 (-912.0696, 276.3895) -> (-906.5704, 276.3895) centre (-909.32, 277.977) ccw
  line L241 (-899.3696, 288.8615) -> (-906.5704, 276.3895)
  line L242 (-916.5207, 293.624) -> (-902.1193, 293.624)
  arc A237 (-906.7631, 268.5167) -> (-912.2623, 268.5167) centre (-909.5127, 266.9292) ccw
  line L243 (-899.5623, 256.0447) -> (-906.7631, 268.5167)
  line L244 (-912.2623, 268.5167) -> (-919.4631, 256.0447)
  arc A238 (-919.4631, 256.0447) -> (-916.7134, 251.2822) centre (-916.7134, 254.4572) ccw
  line L245 (-916.7134, 251.2822) -> (-902.312, 251.2822)
  arc A239 (-902.312, 251.2822) -> (-899.5623, 256.0447) centre (-902.312, 254.4572) ccw
  line L246 (-912.0696, 330.7455) -> (-919.2704, 343.2175)
  arc A240 (-899.3696, 343.2175) -> (-902.1193, 347.98) centre (-902.1193, 344.805) ccw
  arc A241 (-916.5207, 347.98) -> (-919.2704, 343.2175) centre (-916.5207, 344.805) ccw
  arc A242 (-912.0696, 330.7455) -> (-906.5704, 330.7455) centre (-909.32, 332.333) ccw
  line L247 (-899.3696, 343.2175) -> (-906.5704, 330.7455)
  line L248 (-916.5207, 347.98) -> (-902.1193, 347.98)
  arc A243 (-906.7631, 322.8727) -> (-912.2623, 322.8727) centre (-909.5127, 321.2852) ccw
  line L249 (-899.5623, 310.4007) -> (-906.7631, 322.8727)
  line L250 (-912.2623, 322.8727) -> (-919.4631, 310.4007)
  arc A244 (-919.4631, 310.4007) -> (-916.7134, 305.6382) centre (-916.7134, 308.8132) ccw
  line L251 (-916.7134, 305.6382) -> (-902.312, 305.6382)
  arc A245 (-902.312, 305.6382) -> (-899.5623, 310.4007) centre (-902.312, 308.8132) ccw
  line L252 (-912.0696, 385.1015) -> (-919.2704, 397.5735)
  arc A246 (-899.3696, 397.5735) -> (-902.1193, 402.336) centre (-902.1193, 399.161) ccw
  arc A247 (-916.5207, 402.336) -> (-919.2704, 397.5735) centre (-916.5207, 399.161) ccw
  arc A248 (-912.0696, 385.1015) -> (-906.5704, 385.1015) centre (-909.32, 386.689) ccw
  line L253 (-899.3696, 397.5735) -> (-906.5704, 385.1015)
  line L254 (-916.5207, 402.336) -> (-902.1193, 402.336)
  arc A249 (-906.7631, 377.2287) -> (-912.2623, 377.2287) centre (-909.5127, 375.6412) ccw
  line L255 (-899.5623, 364.7567) -> (-906.7631, 377.2287)
  line L256 (-912.2623, 377.2287) -> (-919.4631, 364.7567)
  arc A250 (-919.4631, 364.7567) -> (-916.7134, 359.9942) centre (-916.7134, 363.1692) ccw
  line L257 (-916.7134, 359.9942) -> (-902.312, 359.9942)
  arc A251 (-902.312, 359.9942) -> (-899.5623, 364.7567) centre (-902.312, 363.1692) ccw
  line L258 (-857.7136, 58.9655) -> (-864.9144, 71.4375)
  arc A252 (-845.0136, 71.4375) -> (-847.7633, 76.2) centre (-847.7633, 73.025) ccw
  arc A253 (-862.1647, 76.2) -> (-864.9144, 71.4375) centre (-862.1647, 73.025) ccw
  arc A254 (-857.7136, 58.9655) -> (-852.2144, 58.9655) centre (-854.964, 60.553) ccw
  line L259 (-845.0136, 71.4375) -> (-852.2144, 58.9655)
  line L260 (-862.1647, 76.2) -> (-847.7633, 76.2)
  arc A255 (-852.4071, 51.0927) -> (-857.9063, 51.0927) centre (-855.1567, 49.5052) ccw
  line L261 (-845.2063, 38.6207) -> (-852.4071, 51.0927)
  line L262 (-857.9063, 51.0927) -> (-865.1071, 38.6207)
  arc A256 (-865.1071, 38.6207) -> (-862.3574, 33.8582) centre (-862.3574, 37.0332) ccw
  line L263 (-862.3574, 33.8582) -> (-847.956, 33.8582)
  arc A257 (-847.956, 33.8582) -> (-845.2063, 38.6207) centre (-847.956, 37.0332) ccw
  line L264 (-857.7136, 113.3215) -> (-864.9144, 125.7935)
  arc A258 (-845.0136, 125.7935) -> (-847.7633, 130.556) centre (-847.7633, 127.381) ccw
  arc A259 (-862.1647, 130.556) -> (-864.9144, 125.7935) centre (-862.1647, 127.381) ccw
  arc A260 (-857.7136, 113.3215) -> (-852.2144, 113.3215) centre (-854.964, 114.909) ccw
  line L265 (-845.0136, 125.7935) -> (-852.2144, 113.3215)
  line L266 (-862.1647, 130.556) -> (-847.7633, 130.556)
  arc A261 (-852.4071, 105.4487) -> (-857.9063, 105.4487) centre (-855.1567, 103.8612) ccw
  line L267 (-845.2063, 92.9767) -> (-852.4071, 105.4487)
  line L268 (-857.9063, 105.4487) -> (-865.1071, 92.9767)
  arc A262 (-865.1071, 92.9767) -> (-862.3574, 88.2142) centre (-862.3574, 91.3892) ccw
  line L269 (-862.3574, 88.2142) -> (-847.956, 88.2142)
  arc A263 (-847.956, 88.2142) -> (-845.2063, 92.9767) centre (-847.956, 91.3892) ccw
  line L270 (-857.7136, 167.6775) -> (-864.9144, 180.1495)
  arc A264 (-845.0136, 180.1495) -> (-847.7633, 184.912) centre (-847.7633, 181.737) ccw
  arc A265 (-862.1647, 184.912) -> (-864.9144, 180.1495) centre (-862.1647, 181.737) ccw
  arc A266 (-857.7136, 167.6775) -> (-852.2144, 167.6775) centre (-854.964, 169.265) ccw
  line L271 (-845.0136, 180.1495) -> (-852.2144, 167.6775)
  line L272 (-862.1647, 184.912) -> (-847.7633, 184.912)
  arc A267 (-852.4071, 159.8047) -> (-857.9063, 159.8047) centre (-855.1567, 158.2172) ccw
  line L273 (-845.2063, 147.3327) -> (-852.4071, 159.8047)
  line L274 (-857.9063, 159.8047) -> (-865.1071, 147.3327)
  arc A268 (-865.1071, 147.3327) -> (-862.3574, 142.5702) centre (-862.3574, 145.7452) ccw
  line L275 (-862.3574, 142.5702) -> (-847.956, 142.5702)
  arc A269 (-847.956, 142.5702) -> (-845.2063, 147.3327) centre (-847.956, 145.7452) ccw
  line L276 (-857.7136, 222.0335) -> (-864.9144, 234.5055)
  arc A270 (-845.0136, 234.5055) -> (-847.7633, 239.268) centre (-847.7633, 236.093) ccw
  arc A271 (-862.1647, 239.268) -> (-864.9144, 234.5055) centre (-862.1647, 236.093) ccw
  arc A272 (-857.7136, 222.0335) -> (-852.2144, 222.0335) centre (-854.964, 223.621) ccw
  line L277 (-845.0136, 234.5055) -> (-852.2144, 222.0335)
  line L278 (-862.1647, 239.268) -> (-847.7633, 239.268)
  arc A273 (-852.4071, 214.1607) -> (-857.9063, 214.1607) centre (-855.1567, 212.5732) ccw
  line L279 (-845.2063, 201.6887) -> (-852.4071, 214.1607)
  line L280 (-857.9063, 214.1607) -> (-865.1071, 201.6887)
  arc A274 (-865.1071, 201.6887) -> (-862.3574, 196.9262) centre (-862.3574, 200.1012) ccw
  line L281 (-862.3574, 196.9262) -> (-847.956, 196.9262)
  arc A275 (-847.956, 196.9262) -> (-845.2063, 201.6887) centre (-847.956, 200.1012) ccw
  line L282 (-857.7136, 276.3895) -> (-864.9144, 288.8615)
  arc A276 (-845.0136, 288.8615) -> (-847.7633, 293.624) centre (-847.7633, 290.449) ccw
  arc A277 (-862.1647, 293.624) -> (-864.9144, 288.8615) centre (-862.1647, 290.449) ccw
  arc A278 (-857.7136, 276.3895) -> (-852.2144, 276.3895) centre (-854.964, 277.977) ccw
  line L283 (-845.0136, 288.8615) -> (-852.2144, 276.3895)
  line L284 (-862.1647, 293.624) -> (-847.7633, 293.624)
  arc A279 (-852.4071, 268.5167) -> (-857.9063, 268.5167) centre (-855.1567, 266.9292) ccw
  line L285 (-845.2063, 256.0447) -> (-852.4071, 268.5167)
  line L286 (-857.9063, 268.5167) -> (-865.1071, 256.0447)
  arc A280 (-865.1071, 256.0447) -> (-862.3574, 251.2822) centre (-862.3574, 254.4572) ccw
  line L287 (-862.3574, 251.2822) -> (-847.956, 251.2822)
  arc A281 (-847.956, 251.2822) -> (-845.2063, 256.0447) centre (-847.956, 254.4572) ccw
  line L288 (-857.7136, 330.7455) -> (-864.9144, 343.2175)
  arc A282 (-845.0136, 343.2175) -> (-847.7633, 347.98) centre (-847.7633, 344.805) ccw
  arc A283 (-862.1647, 347.98) -> (-864.9144, 343.2175) centre (-862.1647, 344.805) ccw
  arc A284 (-857.7136, 330.7455) -> (-852.2144, 330.7455) centre (-854.964, 332.333) ccw
  line L289 (-845.0136, 343.2175) -> (-852.2144, 330.7455)
  line L290 (-862.1647, 347.98) -> (-847.7633, 347.98)
  arc A285 (-852.4071, 322.8727) -> (-857.9063, 322.8727) centre (-855.1567, 321.2852) ccw
  line L291 (-845.2063, 310.4007) -> (-852.4071, 322.8727)
  line L292 (-857.9063, 322.8727) -> (-865.1071, 310.4007)
  arc A286 (-865.1071, 310.4007) -> (-862.3574, 305.6382) centre (-862.3574, 308.8132) ccw
  line L293 (-862.3574, 305.6382) -> (-847.956, 305.6382)
  arc A287 (-847.956, 305.6382) -> (-845.2063, 310.4007) centre (-847.956, 308.8132) ccw
  line L294 (-857.7136, 385.1015) -> (-864.9144, 397.5735)
  arc A288 (-845.0136, 397.5735) -> (-847.7633, 402.336) centre (-847.7633, 399.161) ccw
  arc A289 (-862.1647, 402.336) -> (-864.9144, 397.5735) centre (-862.1647, 399.161) ccw
  arc A290 (-857.7136, 385.1015) -> (-852.2144, 385.1015) centre (-854.964, 386.689) ccw
  line L295 (-845.0136, 397.5735) -> (-852.2144, 385.1015)
  line L296 (-862.1647, 402.336) -> (-847.7633, 402.336)
  arc A291 (-852.4071, 377.2287) -> (-857.9063, 377.2287) centre (-855.1567, 375.6412) ccw
  line L297 (-845.2063, 364.7567) -> (-852.4071, 377.2287)
  line L298 (-857.9063, 377.2287) -> (-865.1071, 364.7567)
  arc A292 (-865.1071, 364.7567) -> (-862.3574, 359.9942) centre (-862.3574, 363.1692) ccw
  line L299 (-862.3574, 359.9942) -> (-847.956, 359.9942)
  arc A293 (-847.956, 359.9942) -> (-845.2063, 364.7567) centre (-847.956, 363.1692) ccw
  line L300 (-803.3576, 58.9655) -> (-810.5584, 71.4375)
  arc A294 (-790.6576, 71.4375) -> (-793.4073, 76.2) centre (-793.4073, 73.025) ccw
  arc A295 (-807.8087, 76.2) -> (-810.5584, 71.4375) centre (-807.8087, 73.025) ccw
  arc A296 (-803.3576, 58.9655) -> (-797.8584, 58.9655) centre (-800.608, 60.553) ccw
  line L301 (-790.6576, 71.4375) -> (-797.8584, 58.9655)
  line L302 (-807.8087, 76.2) -> (-793.4073, 76.2)
  arc A297 (-798.0511, 51.0927) -> (-803.5503, 51.0927) centre (-800.8007, 49.5052) ccw
  line L303 (-790.8503, 38.6207) -> (-798.0511, 51.0927)
  line L304 (-803.5503, 51.0927) -> (-810.7511, 38.6207)
  arc A298 (-810.7511, 38.6207) -> (-808.0014, 33.8582) centre (-808.0014, 37.0332) ccw
  line L305 (-808.0014, 33.8582) -> (-793.6, 33.8582)
  arc A299 (-793.6, 33.8582) -> (-790.8503, 38.6207) centre (-793.6, 37.0332) ccw
  line L306 (-803.3576, 113.3215) -> (-810.5584, 125.7935)
  arc A300 (-790.6576, 125.7935) -> (-793.4073, 130.556) centre (-793.4073, 127.381) ccw
  arc A301 (-807.8087, 130.556) -> (-810.5584, 125.7935) centre (-807.8087, 127.381) ccw
  arc A302 (-803.3576, 113.3215) -> (-797.8584, 113.3215) centre (-800.608, 114.909) ccw
  line L307 (-790.6576, 125.7935) -> (-797.8584, 113.3215)
  line L308 (-807.8087, 130.556) -> (-793.4073, 130.556)
  arc A303 (-798.0511, 105.4487) -> (-803.5503, 105.4487) centre (-800.8007, 103.8612) ccw
  line L309 (-790.8503, 92.9767) -> (-798.0511, 105.4487)
  line L310 (-803.5503, 105.4487) -> (-810.7511, 92.9767)
  arc A304 (-810.7511, 92.9767) -> (-808.0014, 88.2142) centre (-808.0014, 91.3892) ccw
  line L311 (-808.0014, 88.2142) -> (-793.6, 88.2142)
  arc A305 (-793.6, 88.2142) -> (-790.8503, 92.9767) centre (-793.6, 91.3892) ccw
  line L312 (-803.3576, 167.6775) -> (-810.5584, 180.1495)
  arc A306 (-790.6576, 180.1495) -> (-793.4073, 184.912) centre (-793.4073, 181.737) ccw
  arc A307 (-807.8087, 184.912) -> (-810.5584, 180.1495) centre (-807.8087, 181.737) ccw
  arc A308 (-803.3576, 167.6775) -> (-797.8584, 167.6775) centre (-800.608, 169.265) ccw
  line L313 (-790.6576, 180.1495) -> (-797.8584, 167.6775)
  line L314 (-807.8087, 184.912) -> (-793.4073, 184.912)
  arc A309 (-798.0511, 159.8047) -> (-803.5503, 159.8047) centre (-800.8007, 158.2172) ccw
  line L315 (-790.8503, 147.3327) -> (-798.0511, 159.8047)
  line L316 (-803.5503, 159.8047) -> (-810.7511, 147.3327)
  arc A310 (-810.7511, 147.3327) -> (-808.0014, 142.5702) centre (-808.0014, 145.7452) ccw
  line L317 (-808.0014, 142.5702) -> (-793.6, 142.5702)
  arc A311 (-793.6, 142.5702) -> (-790.8503, 147.3327) centre (-793.6, 145.7452) ccw
  line L318 (-803.3576, 222.0335) -> (-810.5584, 234.5055)
  arc A312 (-790.6576, 234.5055) -> (-793.4073, 239.268) centre (-793.4073, 236.093) ccw
  arc A313 (-807.8087, 239.268) -> (-810.5584, 234.5055) centre (-807.8087, 236.093) ccw
  arc A314 (-803.3576, 222.0335) -> (-797.8584, 222.0335) centre (-800.608, 223.621) ccw
  line L319 (-790.6576, 234.5055) -> (-797.8584, 222.0335)
  line L320 (-807.8087, 239.268) -> (-793.4073, 239.268)
  arc A315 (-798.0511, 214.1607) -> (-803.5503, 214.1607) centre (-800.8007, 212.5732) ccw
  line L321 (-790.8503, 201.6887) -> (-798.0511, 214.1607)
  line L322 (-803.5503, 214.1607) -> (-810.7511, 201.6887)
  arc A316 (-810.7511, 201.6887) -> (-808.0014, 196.9262) centre (-808.0014, 200.1012) ccw
  line L323 (-808.0014, 196.9262) -> (-793.6, 196.9262)
  arc A317 (-793.6, 196.9262) -> (-790.8503, 201.6887) centre (-793.6, 200.1012) ccw
  line L324 (-803.3576, 276.3895) -> (-810.5584, 288.8615)
  arc A318 (-790.6576, 288.8615) -> (-793.4073, 293.624) centre (-793.4073, 290.449) ccw
  arc A319 (-807.8087, 293.624) -> (-810.5584, 288.8615) centre (-807.8087, 290.449) ccw
  arc A320 (-803.3576, 276.3895) -> (-797.8584, 276.3895) centre (-800.608, 277.977) ccw
  line L325 (-790.6576, 288.8615) -> (-797.8584, 276.3895)
  line L326 (-807.8087, 293.624) -> (-793.4073, 293.624)
  arc A321 (-798.0511, 268.5167) -> (-803.5503, 268.5167) centre (-800.8007, 266.9292) ccw
  line L327 (-790.8503, 256.0447) -> (-798.0511, 268.5167)
  line L328 (-803.5503, 268.5167) -> (-810.7511, 256.0447)
  arc A322 (-810.7511, 256.0447) -> (-808.0014, 251.2822) centre (-808.0014, 254.4572) ccw
  line L329 (-808.0014, 251.2822) -> (-793.6, 251.2822)
  arc A323 (-793.6, 251.2822) -> (-790.8503, 256.0447) centre (-793.6, 254.4572) ccw
  line L330 (-803.3576, 330.7455) -> (-810.5584, 343.2175)
  arc A324 (-790.6576, 343.2175) -> (-793.4073, 347.98) centre (-793.4073, 344.805) ccw
  arc A325 (-807.8087, 347.98) -> (-810.5584, 343.2175) centre (-807.8087, 344.805) ccw
  arc A326 (-803.3576, 330.7455) -> (-797.8584, 330.7455) centre (-800.608, 332.333) ccw
  line L331 (-790.6576, 343.2175) -> (-797.8584, 330.7455)
  line L332 (-807.8087, 347.98) -> (-793.4073, 347.98)